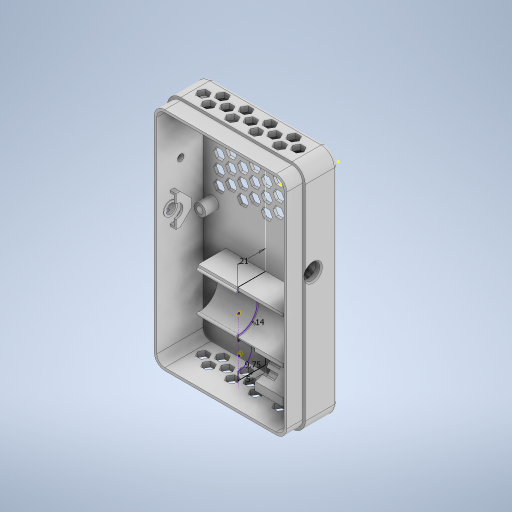
# Autodesk Inventor part: Bottom Housing
Saved by Autodesk Inventor 2023 (Build 270158000, 158)
## iProperties
Created: 2024-03-20
Part Number: Bottom Housing
Material: Generic
Document SubType Name: Modeling
Designer: Pobe Tran
Density: 1 g/cm^3
Appearance: Default
Author: Pobe Tran
Autodesk Inventor part; units mm, degrees
(part 1 of 2)
sketch "Sketch2" plane through (0, 0, 0) normal (0, 0, 1) x (1, 0, 0)
  line L0 (0, 0) -> (-90.043, 0)
  line L1 (-90.043, 0) -> (-90.043, -76.2)
  line L2 (-90.043, -76.2) -> (0, -76.2)
  line L3 (0, -76.2) -> (0, 0)
  circle A0 centre (-6.858, -17.272) radius 0.45
  circle A1 centre (-11.938, -17.272) radius 0.45
  circle A2 centre (-9.398, -17.272) radius 0.45
  circle A3 centre (-9.398, -35.052) radius 0.45
  circle A4 centre (-6.858, -35.052) radius 0.45
  circle A5 centre (-14.478, -17.272) radius 0.45
  circle A6 centre (-14.478, -35.052) radius 0.45
  circle A7 centre (-17.018, -17.272) radius 0.45
  circle A8 centre (-22.098, -17.272) radius 0.45
  circle A9 centre (-19.558, -17.272) radius 0.45
  circle A10 centre (-27.178, -17.272) radius 0.45
  circle A11 centre (-24.638, -17.272) radius 0.45
  circle A12 centre (-29.718, -17.272) radius 0.45
  circle A13 centre (-29.718, -35.052) radius 0.45
  circle A14 centre (-4.445, -46.736) radius 0.55
  circle A15 centre (-11.938, -35.052) radius 0.45
  circle A16 centre (-4.445, -44.196) radius 0.55
  circle A17 centre (-4.445, -49.276) radius 0.55
  line L4 (-11.023, -61.594) -> (-11.023, -64.644)
  line L5 (-10.263, -61.594) -> (-11.023, -61.594)
  line L6 (-10.263, -64.644) -> (-10.263, -61.594)
  line L7 (-11.023, -64.644) -> (-10.263, -64.644)
  line L8 (-14.498, -58.009) -> (-14.498, -58.769)
  line L9 (-11.448, -58.009) -> (-14.498, -58.009)
  line L10 (-11.448, -58.769) -> (-11.448, -58.009)
  line L11 (-14.498, -58.769) -> (-11.448, -58.769)
  line L12 (-16.953, -61.594) -> (-16.953, -64.644)
  line L13 (-16.193, -61.594) -> (-16.953, -61.594)
  line L14 (-16.193, -64.644) -> (-16.193, -61.594)
  line L15 (-16.953, -64.644) -> (-16.193, -64.644)
  circle A18 centre (-17.018, -35.052) radius 0.45
  circle A19 centre (-22.098, -35.052) radius 0.45
  circle A20 centre (-19.558, -35.052) radius 0.45
  circle A21 centre (-27.178, -35.052) radius 0.45
  circle A22 centre (-24.638, -35.052) radius 0.45
  circle A23 centre (-28.067, -58.036) radius 0.35
  circle A24 centre (-28.067, -65.662) radius 0.35
  circle A25 centre (-32.258, -17.272) radius 0.45
  circle A26 centre (-37.338, -17.272) radius 0.45
  circle A27 centre (-34.798, -17.272) radius 0.45
  circle A28 centre (-37.338, -35.052) radius 0.45
  circle A29 centre (-32.258, -35.052) radius 0.45
  circle A30 centre (-39.878, -17.272) radius 0.45
  circle A31 centre (-39.878, -35.052) radius 0.45
  circle A32 centre (-42.418, -17.272) radius 0.45
  circle A33 centre (-47.498, -17.272) radius 0.45
  circle A34 centre (-44.958, -17.272) radius 0.45
  circle A35 centre (-52.578, -17.272) radius 0.45
  circle A36 centre (-50.038, -17.272) radius 0.45
  circle A37 centre (-55.118, -17.272) radius 0.45
  circle A38 centre (-52.578, -35.052) radius 0.45
  circle A39 centre (-34.798, -35.052) radius 0.45
  circle A40 centre (-44.958, -35.052) radius 0.45
  circle A41 centre (-42.418, -35.052) radius 0.45
  circle A42 centre (-32.893, -61.595) radius 0.55
  circle A43 centre (-32.893, -64.135) radius 0.55
  circle A44 centre (-46.101, -58.036) radius 0.35
  circle A45 centre (-32.893, -59.055) radius 0.55
  circle A46 centre (-47.498, -35.052) radius 0.45
  circle A47 centre (-45.212, -46.355) radius 1.9
  circle A48 centre (-55.118, -35.052) radius 0.45
  circle A49 centre (-50.038, -35.052) radius 0.45
  circle A50 centre (-50.546, -64.135) radius 0.55
  circle A51 centre (-46.101, -65.662) radius 0.35
  circle A52 centre (-50.546, -59.055) radius 0.55
  circle A53 centre (-50.546, -61.595) radius 0.55
  line L16 (-93.5594, -83.82) -> (-93.5594, 3.4535)
  line L17 (-93.5594, 3.4535) -> (2.8371, 3.4535)
  line L18 (2.8371, 3.4535) -> (2.8371, -113.1572)
  line L19 (2.8371, -113.1572) -> (2.8371, -163.9139)
  line L20 (2.8371, -163.9139) -> (-93.5594, -163.9139)
  line L21 (-93.5594, -163.9139) -> (-93.5594, -83.82)
  constraints: 54 centre point, 44 end point, 2 collinear
extrude "Extrusion2" add sketch "Sketch2" along normal blind 2 contours L3 L2 L1 L0 | A0 | A1 | A2 | A3 | A4 | A5 | A6 | A7 | A8 | A9 | A10 | A11 | A12 | A13 | A14 | A15 | A16 | A17 | L5 L6 L7 L4 | L9 L10 L11 L8 | L13 L14 L15 L12 | A18 | A19 | A20 | A21 | A22 | A23 | A24 | A25 | A26 | A27 | A28 | A29 | A30 | A31 | A32 | A33 | A34 | A35 | A36 | A37 | A38 | A39 | A40 | A41 | A42 | A43 | A44 | A45 | A46 | A47 | A48 | A49 | A50 | A51 | A52 | A53 | L16 L17 L18 L19 L20 L21
sketch "Sketch3" plane through (0, 0, 2) normal (0, 0, 1) x (1, 0, 0)
  line L0 (-90.043, 0) -> (-90.043, -76.2) projected
  line L1 (-90.043, -76.2) -> (0, -76.2) projected
  line L2 (0, -76.2) -> (0, 0) projected
  line L3 (0, 0) -> (-90.043, 0) projected
  circle A0 centre (-4, -72.2) radius 2.45
  circle A1 centre (-4, -4) radius 2.45
  circle A2 centre (-86.043, -72.2) radius 2.45
  circle A3 centre (-86.043, -4) radius 2.45
  circle A4 centre (-4, -72.2) radius 4.45
  circle A5 centre (-86.043, -72.2) radius 4.45
  circle A6 centre (-4, -4) radius 4.45
  circle A7 centre (-86.043, -4) radius 4.45
  dimension "d8" = 4
  dimension "d9" = 4
  dimension "d14" = 4
  dimension "d15" = 4
  dimension "d16" = 4.9
  dimension "d17" = 4.9
  dimension "d18" = 4.9
  dimension "d19" = 4.9
  dimension "d22" = 2
  dimension "d23" = 2
  dimension "d24" = 2
  dimension "d25" = 2
  constraints: 8 centre point, 4 coincident, 2 horizontal alignment, 2 vertical alignment
  measures "d8" distance from line of point (-4, -4) L2
  measures "d9" distance from line of point (-4, -4) L3
  measures "d14" distance from line of point (-4, -72.2) L1
  measures "d15" distance from line of L0 point (-86.043, -72.2)
  measures "d16" diameter of A0
  measures "d17" diameter of A1
  measures "d18" diameter of A2
  measures "d19" diameter of A3
  measures "d22" radial gap between concentric circles of A0 A4
  measures "d23" radial gap between concentric circles of A2 A5
  measures "d24" radial gap between concentric circles of A1 A6
  measures "d25" radial gap between concentric circles of A3 A7
extrude "Extrusion4" add sketch "Sketch3" along normal blind 10 contours A7 L3 L0 | L0 A7 | A7 L3 | A5 L1 L0 | L0 A5 | A6 L3 | L3 A6 L2 | L2 A6 | L1 A5 | A4 L2 | L2 A4 L1 | L1 A4 picked at (-86.1414, -0.5226) picked at (-85.9446, -75.6774) picked at (-3.9016, -0.5226) picked at (-3.9016, -75.6774)
sketch "Sketch4" plane through (0, 0, 2) normal (0, 0, 1) x (1, 0, 0)
  point P0 (0, 0)
sketch "Sketch5" plane through (0, 0, 2) normal (0, 0, 1) x (1, 0, 0)
  line L0 (-20.397, -28.9385) -> (-16.0669, -28.9385)
  line L1 (-16.0669, -28.9385) -> (-13.9018, -32.6885)
  line L2 (-13.9018, -32.6885) -> (-16.0669, -36.4385)
  line L3 (-16.0669, -36.4385) -> (-20.397, -36.4385)
  line L4 (-20.397, -36.4385) -> (-22.5621, -32.6885)
  line L5 (-22.5621, -32.6885) -> (-20.397, -28.9385)
  line L6 (-11.397, -34.35) -> (-7.0669, -34.35)
  line L7 (-7.0669, -34.35) -> (-4.9018, -38.1)
  line L8 (-4.9018, -38.1) -> (-7.0669, -41.85)
  line L9 (-7.0669, -41.85) -> (-11.397, -41.85)
  line L10 (-11.397, -41.85) -> (-13.5621, -38.1)
  line L11 (-13.5621, -38.1) -> (-11.397, -34.35)
  line L12 (-20.397, -18.1154) -> (-16.0669, -18.1154)
  line L13 (-16.0669, -18.1154) -> (-13.9018, -21.8654)
  line L14 (-13.9018, -21.8654) -> (-16.0669, -25.6154)
  line L15 (-16.0669, -25.6154) -> (-20.397, -25.6154)
  line L16 (-20.397, -25.6154) -> (-22.5621, -21.8654)
  line L17 (-22.5621, -21.8654) -> (-20.397, -18.1154)
  line L18 (-11.397, -23.5269) -> (-7.0669, -23.5269)
  line L19 (-7.0669, -23.5269) -> (-4.9018, -27.2769)
  line L20 (-4.9018, -27.2769) -> (-7.0669, -31.0269)
  line L21 (-7.0669, -31.0269) -> (-11.397, -31.0269)
  line L22 (-11.397, -31.0269) -> (-13.5621, -27.2769)
  line L23 (-13.5621, -27.2769) -> (-11.397, -23.5269)
  line L24 (-31.5621, -27.2769) -> (-29.397, -23.5269)
  line L25 (-29.397, -23.5269) -> (-25.0669, -23.5269)
  line L26 (-25.0669, -23.5269) -> (-22.9018, -27.2769)
  line L27 (-29.397, -31.0269) -> (-31.5621, -27.2769)
  line L28 (-22.9018, -27.2769) -> (-25.0669, -31.0269)
  line L29 (-25.0669, -31.0269) -> (-29.397, -31.0269)
  line L30 (-29.397, -34.35) -> (-25.0669, -34.35)
  line L31 (-31.5621, -38.1) -> (-29.397, -34.35)
  line L32 (-29.397, -41.85) -> (-31.5621, -38.1)
  line L33 (-25.0669, -34.35) -> (-22.9018, -38.1)
  line L34 (-25.0669, -41.85) -> (-29.397, -41.85)
  line L35 (-22.9018, -38.1) -> (-25.0669, -41.85)
  line L36 (-38.397, -28.9385) -> (-34.0669, -28.9385)
  line L37 (-34.0669, -28.9385) -> (-31.9018, -32.6885)
  line L38 (-31.9018, -32.6885) -> (-34.0669, -36.4385)
  line L39 (-34.0669, -36.4385) -> (-38.397, -36.4385)
  line L40 (-38.397, -36.4385) -> (-40.5621, -32.6885)
  line L41 (-40.5621, -32.6885) -> (-38.397, -28.9385)
  line L42 (-34.0669, -25.6154) -> (-38.397, -25.6154)
  line L43 (-31.9018, -21.8654) -> (-34.0669, -25.6154)
  line L44 (-34.0669, -18.1154) -> (-31.9018, -21.8654)
  line L45 (-38.397, -25.6154) -> (-40.5621, -21.8654)
  line L46 (-38.397, -18.1154) -> (-34.0669, -18.1154)
  line L47 (-40.5621, -21.8654) -> (-38.397, -18.1154)
  line L48 (-20.397, -50.2615) -> (-16.0669, -50.2615)
  line L49 (-16.0669, -50.2615) -> (-13.9018, -54.0115)
  line L50 (-13.9018, -54.0115) -> (-16.0669, -57.7615)
  line L51 (-16.0669, -57.7615) -> (-20.397, -57.7615)
  line L52 (-20.397, -57.7615) -> (-22.5621, -54.0115)
  line L53 (-22.5621, -54.0115) -> (-20.397, -50.2615)
  line L54 (-11.397, -55.6731) -> (-7.0669, -55.6731)
  line L55 (-7.0669, -55.6731) -> (-4.9018, -59.4231)
  line L56 (-4.9018, -59.4231) -> (-7.0669, -63.1731)
  line L57 (-7.0669, -63.1731) -> (-11.397, -63.1731)
  line L58 (-11.397, -63.1731) -> (-13.5621, -59.4231)
  line L59 (-13.5621, -59.4231) -> (-11.397, -55.6731)
  line L60 (-20.397, -39.4385) -> (-16.0669, -39.4385)
  line L61 (-16.0669, -39.4385) -> (-13.9018, -43.1885)
  line L62 (-13.9018, -43.1885) -> (-16.0669, -46.9385)
  line L63 (-16.0669, -46.9385) -> (-20.397, -46.9385)
  line L64 (-20.397, -46.9385) -> (-22.5621, -43.1885)
  line L65 (-22.5621, -43.1885) -> (-20.397, -39.4385)
  line L66 (-11.397, -44.85) -> (-7.0669, -44.85)
  line L67 (-7.0669, -44.85) -> (-4.9018, -48.6)
  line L68 (-4.9018, -48.6) -> (-7.0669, -52.35)
  line L69 (-7.0669, -52.35) -> (-11.397, -52.35)
  line L70 (-11.397, -52.35) -> (-13.5621, -48.6)
  line L71 (-13.5621, -48.6) -> (-11.397, -44.85)
  line L72 (-31.5621, -48.6) -> (-29.397, -44.85)
  line L73 (-29.397, -44.85) -> (-25.0669, -44.85)
  line L74 (-25.0669, -44.85) -> (-22.9018, -48.6)
  line L75 (-29.397, -52.35) -> (-31.5621, -48.6)
  line L76 (-22.9018, -48.6) -> (-25.0669, -52.35)
  line L77 (-25.0669, -52.35) -> (-29.397, -52.35)
  line L78 (-29.397, -55.6731) -> (-25.0669, -55.6731)
  line L79 (-31.5621, -59.4231) -> (-29.397, -55.6731)
  line L80 (-29.397, -63.1731) -> (-31.5621, -59.4231)
  line L81 (-25.0669, -55.6731) -> (-22.9018, -59.4231)
  line L82 (-25.0669, -63.1731) -> (-29.397, -63.1731)
  line L83 (-22.9018, -59.4231) -> (-25.0669, -63.1731)
  line L84 (-38.397, -50.2615) -> (-34.0669, -50.2615)
  line L85 (-34.0669, -50.2615) -> (-31.9018, -54.0115)
  line L86 (-31.9018, -54.0115) -> (-34.0669, -57.7615)
  line L87 (-34.0669, -57.7615) -> (-38.397, -57.7615)
  line L88 (-38.397, -57.7615) -> (-40.5621, -54.0115)
  line L89 (-40.5621, -54.0115) -> (-38.397, -50.2615)
  line L90 (-34.0669, -46.9385) -> (-38.397, -46.9385)
  line L91 (-31.9018, -43.1885) -> (-34.0669, -46.9385)
  line L92 (-34.0669, -39.4385) -> (-31.9018, -43.1885)
  line L93 (-38.397, -46.9385) -> (-40.5621, -43.1885)
  line L94 (-38.397, -39.4385) -> (-34.0669, -39.4385)
  line L95 (-40.5621, -43.1885) -> (-38.397, -39.4385)
  line L96 (-36.232, -21.8654) -> (-36.232, -54.0115) construction
  line L97 (-52.0669, -28.9385) -> (-56.397, -28.9385)
  line L98 (-56.397, -28.9385) -> (-58.5621, -32.6885)
  line L99 (-58.5621, -32.6885) -> (-56.397, -36.4385)
  line L100 (-56.397, -36.4385) -> (-52.0669, -36.4385)
  line L101 (-52.0669, -36.4385) -> (-49.9018, -32.6885)
  line L102 (-49.9018, -32.6885) -> (-52.0669, -28.9385)
  line L103 (-61.0669, -34.35) -> (-65.397, -34.35)
  line L104 (-65.397, -34.35) -> (-67.5621, -38.1)
  line L105 (-67.5621, -38.1) -> (-65.397, -41.85)
  line L106 (-65.397, -41.85) -> (-61.0669, -41.85)
  line L107 (-61.0669, -41.85) -> (-58.9018, -38.1)
  line L108 (-58.9018, -38.1) -> (-61.0669, -34.35)
  line L109 (-52.0669, -18.1154) -> (-56.397, -18.1154)
  line L110 (-56.397, -18.1154) -> (-58.5621, -21.8654)
  line L111 (-58.5621, -21.8654) -> (-56.397, -25.6154)
  line L112 (-56.397, -25.6154) -> (-52.0669, -25.6154)
  line L113 (-52.0669, -25.6154) -> (-49.9018, -21.8654)
  line L114 (-49.9018, -21.8654) -> (-52.0669, -18.1154)
  line L115 (-61.0669, -23.5269) -> (-65.397, -23.5269)
  line L116 (-65.397, -23.5269) -> (-67.5621, -27.2769)
  line L117 (-67.5621, -27.2769) -> (-65.397, -31.0269)
  line L118 (-65.397, -31.0269) -> (-61.0669, -31.0269)
  line L119 (-61.0669, -31.0269) -> (-58.9018, -27.2769)
  line L120 (-58.9018, -27.2769) -> (-61.0669, -23.5269)
  line L121 (-40.9018, -27.2769) -> (-43.0669, -23.5269)
  line L122 (-43.0669, -23.5269) -> (-47.397, -23.5269)
  line L123 (-47.397, -23.5269) -> (-49.5621, -27.2769)
  line L124 (-43.0669, -31.0269) -> (-40.9018, -27.2769)
  line L125 (-49.5621, -27.2769) -> (-47.397, -31.0269)
  line L126 (-47.397, -31.0269) -> (-43.0669, -31.0269)
  line L127 (-43.0669, -34.35) -> (-47.397, -34.35)
  line L128 (-40.9018, -38.1) -> (-43.0669, -34.35)
  line L129 (-43.0669, -41.85) -> (-40.9018, -38.1)
  line L130 (-47.397, -34.35) -> (-49.5621, -38.1)
  line L131 (-47.397, -41.85) -> (-43.0669, -41.85)
  line L132 (-49.5621, -38.1) -> (-47.397, -41.85)
  line L133 (-52.0669, -50.2615) -> (-56.397, -50.2615)
  line L134 (-56.397, -50.2615) -> (-58.5621, -54.0115)
  line L135 (-65.397, -52.35) -> (-61.0669, -52.35)
  line L136 (-61.0669, -52.35) -> (-58.9018, -48.6)
  line L137 (-67.5621, -48.6) -> (-65.397, -52.35)
  line L138 (-65.397, -44.85) -> (-67.5621, -48.6)
  line L139 (-61.0669, -44.85) -> (-65.397, -44.85)
  line L140 (-58.9018, -48.6) -> (-61.0669, -44.85)
  line L141 (-56.397, -46.9385) -> (-52.0669, -46.9385)
  line L142 (-58.5621, -43.1885) -> (-56.397, -46.9385)
  line L143 (-52.0669, -39.4385) -> (-56.397, -39.4385)
  line L144 (-56.397, -39.4385) -> (-58.5621, -43.1885)
  line L145 (-43.0669, -52.35) -> (-40.9018, -48.6)
  line L146 (-40.9018, -48.6) -> (-43.0669, -44.85)
  line L147 (-43.0669, -55.6731) -> (-47.397, -55.6731)
  line L148 (-47.397, -52.35) -> (-43.0669, -52.35)
  line L149 (-43.0669, -44.85) -> (-47.397, -44.85)
  line L150 (-47.397, -44.85) -> (-49.5621, -48.6)
  line L151 (-49.5621, -48.6) -> (-47.397, -52.35)
  line L152 (-49.9018, -54.0115) -> (-52.0669, -50.2615)
  line L153 (-52.0669, -57.7615) -> (-49.9018, -54.0115)
  line L154 (-52.0669, -46.9385) -> (-49.9018, -43.1885)
  line L155 (-49.9018, -43.1885) -> (-52.0669, -39.4385)
  line L156 (-58.5621, -54.0115) -> (-56.397, -57.7615)
  line L157 (-56.397, -57.7615) -> (-52.0669, -57.7615)
  line L158 (-61.0669, -55.6731) -> (-65.397, -55.6731)
  line L159 (-58.9018, -59.4231) -> (-61.0669, -55.6731)
  line L160 (-61.0669, -63.1731) -> (-58.9018, -59.4231)
  line L161 (-65.397, -55.6731) -> (-67.5621, -59.4231)
  line L162 (-65.397, -63.1731) -> (-61.0669, -63.1731)
  line L163 (-67.5621, -59.4231) -> (-65.397, -63.1731)
  line L164 (-40.9018, -59.4231) -> (-43.0669, -55.6731)
  line L165 (-47.397, -55.6731) -> (-49.5621, -59.4231)
  line L166 (-47.397, -63.1731) -> (-43.0669, -63.1731)
  line L167 (-49.5621, -59.4231) -> (-47.397, -63.1731)
  line L168 (-43.0669, -63.1731) -> (-40.9018, -59.4231)
  line L169 (-63.232, -27.2769) -> (-63.232, -59.4231) construction
  line L170 (-70.0669, -39.4385) -> (-67.9018, -43.1885)
  line L171 (-67.9018, -32.6885) -> (-70.0669, -36.4385)
  line L172 (-74.397, -39.4385) -> (-70.0669, -39.4385)
  line L173 (-70.0669, -36.4385) -> (-74.397, -36.4385)
  line L174 (-74.397, -36.4385) -> (-76.5621, -32.6885)
  line L175 (-76.5621, -43.1885) -> (-74.397, -39.4385)
  line L176 (-67.9018, -43.1885) -> (-70.0669, -46.9385)
  line L177 (-70.0669, -46.9385) -> (-74.397, -46.9385)
  line L178 (-74.397, -50.2615) -> (-70.0669, -50.2615)
  line L179 (-70.0669, -50.2615) -> (-67.9018, -54.0115)
  line L180 (-74.397, -28.9385) -> (-70.0669, -28.9385)
  line L181 (-70.0669, -28.9385) -> (-67.9018, -32.6885)
  line L182 (-76.5621, -32.6885) -> (-74.397, -28.9385)
  line L183 (-74.397, -18.1154) -> (-70.0669, -18.1154)
  line L184 (-70.0669, -18.1154) -> (-67.9018, -21.8654)
  line L185 (-67.9018, -21.8654) -> (-70.0669, -25.6154)
  line L186 (-70.0669, -25.6154) -> (-74.397, -25.6154)
  line L187 (-74.397, -25.6154) -> (-76.5621, -21.8654)
  line L188 (-76.5621, -21.8654) -> (-74.397, -18.1154)
  line L189 (-74.397, -46.9385) -> (-76.5621, -43.1885)
  line L190 (-76.5621, -54.0115) -> (-74.397, -50.2615)
  line L191 (-70.0669, -57.7615) -> (-74.397, -57.7615)
  line L192 (-67.9018, -54.0115) -> (-70.0669, -57.7615)
  line L193 (-74.397, -57.7615) -> (-76.5621, -54.0115)
  line L194 (-76.9018, -38.1) -> (-79.0669, -41.85)
  line L195 (-79.0669, -34.35) -> (-76.9018, -38.1)
  line L196 (-76.9018, -27.2769) -> (-79.0669, -31.0269)
  line L197 (-83.397, -23.5269) -> (-79.0669, -23.5269)
  line L198 (-79.0669, -31.0269) -> (-83.397, -31.0269)
  line L199 (-85.5621, -27.2769) -> (-83.397, -23.5269)
  line L200 (-83.397, -31.0269) -> (-85.5621, -27.2769)
  line L201 (-83.397, -34.35) -> (-79.0669, -34.35)
  line L202 (-85.5621, -38.1) -> (-83.397, -34.35)
  line L203 (-83.397, -41.85) -> (-85.5621, -38.1)
  line L204 (-79.0669, -23.5269) -> (-76.9018, -27.2769)
  line L205 (-79.0669, -41.85) -> (-83.397, -41.85)
  line L206 (-79.0669, -44.85) -> (-76.9018, -48.6)
  line L207 (-76.9018, -48.6) -> (-79.0669, -52.35)
  line L208 (-83.397, -44.85) -> (-79.0669, -44.85)
  line L209 (-79.0669, -52.35) -> (-83.397, -52.35)
  line L210 (-85.5621, -48.6) -> (-83.397, -44.85)
  line L211 (-83.397, -52.35) -> (-85.5621, -48.6)
  line L212 (-76.9018, -59.4231) -> (-79.0669, -63.1731)
  line L213 (-79.0669, -55.6731) -> (-76.9018, -59.4231)
  line L214 (-83.397, -55.6731) -> (-79.0669, -55.6731)
  line L215 (-85.5621, -59.4231) -> (-83.397, -55.6731)
  line L216 (-83.397, -63.1731) -> (-85.5621, -59.4231)
  line L217 (-79.0669, -63.1731) -> (-83.397, -63.1731)
  line L218 (-72.232, -21.8654) -> (-18.232, -21.8654) construction
  line L219 (-11.397, -20.2038) -> (-7.0669, -20.2038)
  line L220 (-7.0669, -20.2038) -> (-4.9018, -16.4538)
  line L221 (-4.9018, -16.4538) -> (-7.0669, -12.7038)
  line L222 (-7.0669, -12.7038) -> (-11.397, -12.7038)
  line L223 (-11.397, -12.7038) -> (-13.5621, -16.4538)
  line L224 (-13.5621, -16.4538) -> (-11.397, -20.2038)
  line L225 (-31.5621, -16.4538) -> (-29.397, -20.2038)
  line L226 (-29.397, -20.2038) -> (-25.0669, -20.2038)
  line L227 (-25.0669, -20.2038) -> (-22.9018, -16.4538)
  line L228 (-29.397, -12.7038) -> (-31.5621, -16.4538)
  line L229 (-22.9018, -16.4538) -> (-25.0669, -12.7038)
  line L230 (-25.0669, -12.7038) -> (-29.397, -12.7038)
  line L231 (-49.5621, -16.4538) -> (-47.397, -12.7038)
  line L232 (-43.0669, -20.2038) -> (-47.397, -20.2038)
  line L233 (-47.397, -12.7038) -> (-43.0669, -12.7038)
  line L234 (-40.9018, -16.4538) -> (-43.0669, -20.2038)
  line L235 (-43.0669, -12.7038) -> (-40.9018, -16.4538)
  line L236 (-47.397, -20.2038) -> (-49.5621, -16.4538)
  line L237 (-61.0669, -12.7038) -> (-58.9018, -16.4538)
  line L238 (-58.9018, -16.4538) -> (-61.0669, -20.2038)
  line L239 (-65.397, -12.7038) -> (-61.0669, -12.7038)
  line L240 (-61.0669, -20.2038) -> (-65.397, -20.2038)
  line L241 (-65.397, -20.2038) -> (-67.5621, -16.4538)
  line L242 (-67.5621, -16.4538) -> (-65.397, -12.7038)
  line L243 (-63.232, -16.4538) -> (-63.232, 15.6923) construction
  line L244 (-79.0669, -20.2038) -> (-76.9018, -16.4538)
  line L245 (-76.9018, -16.4538) -> (-79.0669, -12.7038)
  line L246 (-83.397, -20.2038) -> (-79.0669, -20.2038)
  line L247 (-85.5621, -16.4538) -> (-83.397, -20.2038)
  line L248 (-83.397, -12.7038) -> (-85.5621, -16.4538)
  line L249 (-79.0669, -12.7038) -> (-83.397, -12.7038)
  line L250 (-81.232, -38.1) -> (-9.232, -38.1) construction
  circle A0 centre (-86.043, -4) radius 2.45 construction
  circle A1 centre (-86.043, -72.2) radius 2.45 construction
  line L251 (-86.043, -4) -> (-86.043, -72.2) construction
  line L252 (-86.043, -4) -> (-4.4209, -4) construction
  line L253 (-45.232, -16.4538) -> (-45.232, -59.4231) construction
  point P0 (0, 0)
  point P1 (-18.232, -32.6885)
  point P2 (-9.232, -27.2769)
  point P3 (-27.232, -38.1)
  point P4 (-27.232, -27.2769)
  point P5 (-36.232, -32.6885)
  point P6 (-18.232, -54.0115)
  point P7 (-9.232, -59.4231)
  point P8 (-18.232, -43.1885)
  point P9 (-9.232, -48.6)
  point P10 (-27.232, -59.4231)
  point P11 (-27.232, -48.6)
  point P12 (-36.232, -43.1885)
  point P13 (-54.232, -32.6885)
  point P14 (-63.232, -38.1)
  point P15 (-54.232, -21.8654)
  point P16 (-45.232, -38.1)
  point P17 (-45.232, -27.2769)
  point P18 (-63.232, -48.6)
  point P19 (-54.232, -43.1885)
  point P20 (-45.232, -48.6)
  point P21 (-54.232, -54.0115)
  point P22 (-72.232, -43.1885)
  point P23 (-72.232, -32.6885)
  point P24 (-72.232, -54.0115)
  point P25 (-81.232, -27.2769)
  point P26 (-81.232, -48.6)
  point P27 (-81.232, -59.4231)
  point P28 (-9.232, -16.4538)
  point P29 (-27.232, -16.4538)
  point P30 (-81.232, -16.4538)
  point P31 (-86.043, -38.1)
  point P32 (-45.232, -4)
  dimension "d28" = 7.5
  dimension "d29" = 7.5
  dimension "d30" = 3
  dimension "d31" = 7.5
  dimension "d32" = 7.5
  dimension "d33" = 3
  dimension "d34" = 3
  dimension "d37" = 18
  dimension "d42" = 3
  dimension "d43" = 3
  dimension "d48" = 7.5
  dimension "d49" = 7.5
  dimension "d50" = 3
  dimension "d51" = 7.5
  dimension "d52" = 7.5
  dimension "d53" = 3
  dimension "d54" = 3
  dimension "d55" = 18
  dimension "d56" = 3
  dimension "d57" = 3
  dimension "d59" = 3
  constraints: 508 end point, 176 symmetric about line, 4 vertical alignment, 3 horizontal, 2 collinear, 2 midpoint, 2 vertical, 206 other
  measures "d28" distance between parallel lines of L0 L3
  measures "d29" distance between parallel lines of L6 L9
  measures "d30" distance between parallel lines of L2 L11
  measures "d31" distance between parallel lines of L12 L15
  measures "d32" distance between parallel lines of L18 L21
  measures "d33" distance between parallel lines of L14 L23
  measures "d34" distance between parallel lines of L22 L1
  measures "d37" distance of L250.end point (-27.232, -38.1)
  measures "d42" distance between parallel lines of L5 L28
  measures "d43" distance between parallel lines of L4 L33
  measures "d48" distance between parallel lines of L48 L51
  measures "d49" distance between parallel lines of L54 L57
  measures "d50" distance between parallel lines of L50 L59
  measures "d51" distance between parallel lines of L60 L63
  measures "d52" distance between parallel lines of L66 L69
  measures "d53" distance between parallel lines of L62 L71
  measures "d54" distance between parallel lines of L70 L49
  measures "d55" distance of point (-9.232, -59.423) point (-27.232, -59.423)
  measures "d56" distance between parallel lines of L53 L76
  measures "d57" distance between parallel lines of L52 L81
  measures "d59" distance of L67.start L8.end
extrude "Extrusion5" cut sketch "Sketch5" against normal through all
ref_plane "Work Plane5" through (-18.3368, -95.497, 22.3224) normal (1, 0, 0) x (0, -0.4604848, 0.8876676)
sketch "Sketch7" plane through (-18.3368, -95.497, 22.3224) normal (1, 0, 0) x (0, -0.4604848, 0.8876676)
  line L0 (-63.6047, -78.477) -> (13.4654, 70.0896) projected
  line L1 (-11.115, 22.7064) -> (-25.6416, -5.2963)
  line L2 (-11.115, 22.7064) -> (-25.3738, -4.78)
  line L3 (13.4654, 70.0896) -> (-63.6047, -78.477) projected
  line L4 (17.6699, 32.5904) -> (-0.9711, 42.2606)
  line L5 (-11.115, 22.7064) -> (-9.776, 25.2876)
  line L6 (1.5185, 1.4556) -> (-17.1225, 11.1258)
  line L7 (-25.3738, -4.78) -> (-17.1225, 11.1258)
  arc A0 (16.6327, 30.591) -> (2.5557, 3.455) centre (8.9927, 17.335) ccw
  line L8 (1.5185, 1.4556) -> (2.5557, 3.455)
  line L9 (11.6901, 71.0106) -> (13.4654, 70.0896) projected
  line L10 (17.6699, 32.5904) -> (16.6327, 30.591)
  line L11 (8.9927, 17.335) -> (14.927, 28.7745) construction
  circle A1 centre (8.9927, 17.335) radius 1.5875 projected
  circle A2 centre (8.9927, 17.335) radius 15.3 projected
  circle A3 centre (8.9927, 17.335) radius 14 projected
  point P0 (-63.7898, -74.4905)
  point P1 (22.9456, 11.0577)
  point P2 (22.1601, 9.5434)
  point P3 (-21.2482, 3.1729)
  point P4 (-17.1225, 11.1258)
  point P5 (-0.9711, 42.2606)
  point P6 (12.5777, 70.5501)
  dimension "d71" = 35.0748
  dimension "d159" = 15.3
  dimension "d160" = 21
  constraints: 18 end point, 7 point on line, 4 point on circle, 3 parallel, 2 equal length, 2 midpoint, 2 perpendicular, 1 centre point, 1 collinear
  measures "d71" distance between parallel lines of L6 L4
  measures "d159" radius of A0
  measures "d160" distance between parallel lines of L2 L8
extrude "Extrusion6" add sketch "Sketch7" along normal blind 5 and the other way blind 28 contours L0 L4 L10 A0 L8 L6
sketch "Sketch8" plane through (-46.3368, -95.497, 22.3224) normal (-1, 0, 0) x (0, -0.4604848, 0.8876676)
  line L0 (-63.6047, 78.477) -> (13.4654, -70.0896) projected
  line L1 (3.1465, -4.5939) -> (1.5185, -1.4556)
  line L2 (-17.1225, -11.1258) -> (1.5185, -1.4556) projected
  line L3 (1.5185, -1.4556) -> (-17.1225, -11.1258)
  line L4 (-17.1225, -11.1258) -> (11.163, -65.6513)
  arc A0 (3.1465, -4.5939) -> (16.0254, -29.4204) centre (8.9946, -17.3139) ccw
  line L5 (29.804, -55.9811) -> (11.163, -65.6513)
  line L6 (16.0254, -29.4204) -> (18.0003, -33.2273)
  line L7 (26.9588, -50.4963) -> (29.804, -55.9811)
  arc A1 (18.0003, -33.2273) -> (26.9588, -50.4963) centre (21.8882, -42.1686) ccw
  line L8 (11.6901, -71.0106) -> (13.4654, -70.0896) projected
  line L9 (8.9946, -17.3139) -> (32.3631, -62.3609) construction
  line L10 (16.6327, -30.591) -> (17.6699, -32.5904) projected
  line L11 (17.6699, -32.5904) -> (-0.9711, -42.2606)
  line L12 (17.0129, -31.3238) -> (-1.6282, -40.994)
  circle A2 centre (8.9927, -17.335) radius 1.5875 projected
  ellipse E0 centre (20.7156, -41.9283) end of major axis (20.2797, -43.8802) minor radius 1.9704 projected
  point P0 (-63.7898, 74.4905)
  point P1 (2.8668, -43.144)
  point P2 (-1.6282, -40.994)
  dimension "d79" = 21
  dimension "d161" = 5
  dimension "d162" = 9.75
  dimension "d163" = 14
  constraints: 19 end point, 6 point on line, 4 parallel, 4 point on circle, 3 perpendicular, 2 centre point, 1 coincident, 1 collinear, 1 midpoint, 1 other
  measures "d79" distance between parallel lines of L0 L1
  measures "d161" distance between parallel lines of L5 L8
  measures "d162" radius of A1
  measures "d163" radius of A0
extrude "Extrusion7" add sketch "Sketch8" along normal blind 30 contours L2 L1 A0 L6 L12 L0
sketch "Sketch11" plane through (0, 0, 2) normal (0, 0, 1) x (1, 0, 0)
  line L0 (-93.5594, 3.4535) -> (-93.5594, -163.9139) projected
  line L1 (-87.5594, -167.9139) -> (-3.1629, -167.9139)
  line L2 (6.8371, -157.9139) -> (6.8371, -2.5465)
  line L3 (-3.1629, 7.4535) -> (-87.5594, 7.4535)
  line L4 (-97.5594, -2.5465) -> (-97.5594, -157.9139)
  arc A0 (-97.5594, -157.9139) -> (-87.5594, -167.9139) centre (-87.5594, -157.9139) ccw
  arc A1 (-87.5594, 7.4535) -> (-97.5594, -2.5465) centre (-87.5594, -2.5465) ccw
  arc A2 (-3.1629, -167.9139) -> (6.8371, -157.9139) centre (-3.1629, -157.9139) ccw
  arc A3 (6.8371, -2.5465) -> (-3.1629, 7.4535) centre (-3.1629, -2.5465) ccw
  line L5 (-93.5594, -19.0465) -> (-93.5594, -141.4139)
  line L6 (2.8371, 3.4535) -> (-93.5594, 3.4535) projected
  line L7 (-93.5594, -163.9139) -> (2.8371, -163.9139) projected
  line L8 (2.8371, -163.9139) -> (2.8371, 3.4535) projected
  line L9 (-93.5594, -157.9139) -> (-93.5594, -2.5465)
  arc A4 (-87.5594, 3.4535) -> (-93.5594, -2.5465) centre (-87.5594, -2.5465) ccw
  line L10 (-87.5594, 3.4535) -> (-3.1629, 3.4535)
  arc A5 (2.8371, -2.5465) -> (-3.1629, 3.4535) centre (-3.1629, -2.5465) ccw
  line L11 (2.8371, -2.5465) -> (2.8371, -157.9139)
  arc A6 (-3.1629, -163.9139) -> (2.8371, -157.9139) centre (-3.1629, -157.9139) ccw
  line L12 (-3.1629, -163.9139) -> (-87.5594, -163.9139)
  arc A7 (-93.5594, -157.9139) -> (-87.5594, -163.9139) centre (-87.5594, -157.9139) ccw
  line L13 (-87.5594, -165.9139) -> (-3.1629, -165.9139)
  arc A8 (-3.1629, -165.9139) -> (4.8371, -157.9139) centre (-3.1629, -157.9139) ccw
  line L14 (4.8371, -157.9139) -> (4.8371, -2.5465)
  arc A9 (4.8371, -2.5465) -> (-3.1629, 5.4535) centre (-3.1629, -2.5465) ccw
  line L15 (-3.1629, 5.4535) -> (-87.5594, 5.4535)
  arc A10 (-87.5594, 5.4535) -> (-95.5594, -2.5465) centre (-87.5594, -2.5465) ccw
  line L16 (-95.5594, -2.5465) -> (-95.5594, -157.9139)
  arc A11 (-95.5594, -157.9139) -> (-87.5594, -165.9139) centre (-87.5594, -157.9139) ccw
  point P0 (-97.5594, -167.9139)
  point P1 (6.8371, -167.9139)
  point P2 (6.8371, 7.4535)
  point P3 (-97.5594, 7.4535)
  point P4 (2.8371, -2.5465)
  point P5 (-3.1629, -163.9139)
  point P6 (-87.5594, 3.4535)
  dimension "d97" = 10
  dimension "d113" = 4
  dimension "d114" = 4
  dimension "d115" = 4
  dimension "d116" = 4
  dimension "d117" = 2
  constraints: 26 end point, 24 point on circle, 12 centre point, 9 point on line, 8 tangent, 6 parallel, 3 equal radius, 3 perpendicular, 14 other
  measures "d97" radius of A0
  measures "d113" distance between parallel lines of L0 L4
  measures "d114" distance between parallel lines of L6 L3
  measures "d115" distance between parallel lines of L1 L7
  measures "d116" distance between parallel lines of L2 L8
  measures "d117" radial gap between concentric circles of A0 A11
extrude "Extrusion10" add sketch "Sketch11" along normal blind 35 and the other way blind 2 contours L0 A11 L16 A10 | L0 A10 L6 A4 | L0 L6 A10 | L6 A10 L15 A9 | L6 A9 L8 A5 | A7 L7 A11 L0 | L6 L8 A9 | L8 A9 L14 A8 | A11 L7 L0 | L7 A8 L13 A11 | L8 A8 L7 A6 | L8 L7 A8 | A0 L4 A1 L3 A3 L2 A2 L1
sketch "Sketch14" plane through (0, 0, 37) normal (0, 0, 1) x (1, 0, 0)
  point P0 (0, 0)
sketch "Sketch15" plane through (0, 0, 37) normal (0, 0, 1) x (1, 0, 0)
  arc A0 (-3.1629, -167.9139) -> (6.8371, -157.9139) centre (-3.1629, -157.9139) ccw projected
  line L0 (6.8371, -157.9139) -> (6.8371, -2.5465) projected
  arc A1 (6.8371, -2.5465) -> (-3.1629, 7.4535) centre (-3.1629, -2.5465) ccw projected
  line L1 (-3.1629, 7.4535) -> (-87.5594, 7.4535) projected
  arc A2 (-87.5594, 7.4535) -> (-97.5594, -2.5465) centre (-87.5594, -2.5465) ccw projected
  line L2 (-97.5594, -2.5465) -> (-97.5594, -157.9139) projected
  arc A3 (-97.5594, -157.9139) -> (-87.5594, -167.9139) centre (-87.5594, -157.9139) ccw projected
  line L3 (-87.5594, -167.9139) -> (-3.1629, -167.9139) projected
  line L4 (2.8371, -2.5465) -> (2.8371, -157.9139) projected
  arc A4 (-3.1629, -163.9139) -> (2.8371, -157.9139) centre (-3.1629, -157.9139) ccw projected
  line L5 (-3.1629, -163.9139) -> (-87.5594, -163.9139) projected
  arc A5 (-93.5594, -157.9139) -> (-87.5594, -163.9139) centre (-87.5594, -157.9139) ccw projected
  line L6 (-93.5594, -157.9139) -> (-93.5594, -2.5465) projected
  arc A6 (-87.5594, 3.4535) -> (-93.5594, -2.5465) centre (-87.5594, -2.5465) ccw projected
  line L7 (-87.5594, 3.4535) -> (-3.1629, 3.4535) projected
  arc A7 (2.8371, -2.5465) -> (-3.1629, 3.4535) centre (-3.1629, -2.5465) ccw projected
  line L8 (4.8371, -2.5465) -> (4.8371, -157.9139)
  arc A8 (-3.1629, -165.9139) -> (4.8371, -157.9139) centre (-3.1629, -157.9139) ccw
  line L9 (-3.1629, -165.9139) -> (-87.5594, -165.9139)
  arc A9 (-95.5594, -157.9139) -> (-87.5594, -165.9139) centre (-87.5594, -157.9139) ccw
  line L10 (-95.5594, -157.9139) -> (-95.5594, -2.5465)
  arc A10 (-87.5594, 5.4535) -> (-95.5594, -2.5465) centre (-87.5594, -2.5465) ccw
  line L11 (-87.5594, 5.4535) -> (-3.1629, 5.4535)
  arc A11 (4.8371, -2.5465) -> (-3.1629, 5.4535) centre (-3.1629, -2.5465) ccw
  point P0 (0, 0)
  dimension "d120" = 2
  constraints: 8 end point, 8 point on circle, 4 centre point, 7 other
  measures "d120" distance between parallel lines of L0 L8
extrude "Extrusion12" cut sketch "Sketch15" against normal blind 12
sketch "Sketch16" plane through (6.8371, -157.9139, 0) normal (1, 0, 0) x (0, 0, -1)
  arc A0 (-19.5791, 99.2547) -> (-18.9791, 90.2949) centre (-18.9791, 94.7949) ccw projected
  arc A1 (-17.7544, 96.0449) -> (-17.7544, 93.5449) centre (-18.9791, 94.7949) ccw projected
  circle A2 centre (-18.9791, 94.7949) radius 6
  point P0 (0, 157.9139)
  dimension "d123" = 12
  constraints: 1 centre point, 1 coincident
  measures "d123" diameter of A2
extrude "Extrusion13" cut sketch "Sketch16" against normal up to next
sketch "Sketch17" plane through (-97.5594, -157.9139, 0) normal (-1, 0, 0) x (0, 0, 1)
  circle A0 centre (18.9791, 119.8139) radius 2.5
  line L0 (12.7191, 157.9139) -> (12.7191, 81.7139) projected
  arc A1 (18.9791, 90.2949) -> (19.5791, 99.2547) centre (18.9791, 94.7949) ccw projected
  point P0 (0, 157.9139)
  point P1 (12.7191, 119.8139)
  dimension "d126" = 5
  constraints: 1 centre point, 1 horizontal alignment, 1 midpoint, 1 vertical alignment
  measures "d126" diameter of A0
extrude "Extrusion14" cut sketch "Sketch17" against normal blind 12
chamfer "Chamfer1" distance 1 angle 45 2 edges at (6.8371, -63.119, 24.9791) (-97.5594, -38.1, 16.4791)
fillet "Fillet2" radius 3 8 edges at (3.9082, -164.985, 0) (-45.3611, -167.9139, 0) (-94.6305, -164.985, 0) (-97.5594, -80.2302, 0) (-94.6305, 4.5245, 0) (-45.3611, 7.4535, 0) (3.9082, 4.5245, 0) (6.8371, -80.2302, 0)
sketch "Sketch18" plane through (6.8371, -157.9139, 25) normal (1, 0, 0) x (0, 0, -1)
  point P0 (25, 157.9139)
ref_plane "Work Plane7" through (-78.0651, -167.9139, 25) normal (1, 0, 0) x (0, 1, 0)
sketch "Sketch24" plane through (-78.0651, -167.9139, 25) normal (1, 0, 0) x (0, 1, 0)
  arc A0 (3.175, 26.5) -> (0, 23.325) centre (3.175, 23.325) ccw projected
  line L0 (36.4678, 24.8) -> (36.4678, 23.5) projected
  line L1 (2, 23.5) -> (36.4678, 23.5) projected
  line L2 (2, 0) -> (2, 23.5) projected
  line L3 (0, 0) -> (2, 0) projected
  line L4 (0, 23.325) -> (0, 0) projected
  line L5 (3.175, 26.5) -> (3.175, 24.8) projected
  line L6 (3.175, 24.8) -> (36.4678, 24.8) projected
  point P0 (167.9139, -25)
ref_plane "Work Plane8" through (-12.439, -167.9139, 25) normal (-1, 0, 0) x (0, 0, 1)
extrude "Extrusion20" [suppressed]
sketch "Sketch25" plane through (-78.0651, -131.4461, 51.5) normal (0, 1, 0) x (1, 0, 0)
  point P0 (78.0651, 51.5)
ref_plane "Work Plane9" through (-69.9262, -125.2739, 49.9384) normal (0, -1, 0) x (1, 0, 0)
sketch "Sketch28" plane through (-46.3368, -95.497, 22.3224) normal (1, 0, 0) x (0, 0.4604848, -0.8876676)
  arc A0 (-26.9588, -50.4963) -> (-18.0003, -33.2273) centre (-21.8882, -42.1686) ccw projected
  line L0 (-17.0129, -31.3238) -> (1.6282, -40.994) projected
  line L1 (-16.0254, -29.4204) -> (-18.0003, -33.2273) projected
  line L2 (63.6047, 78.477) -> (-13.4654, -70.0896) projected
  line L3 (-26.9588, -50.4963) -> (-29.804, -55.9811) projected
  line L4 (-29.804, -55.9811) -> (-11.163, -65.6513) projected
  point P0 (63.7898, 74.4905)
extrude "Extrusion24" add sketch "Sketch28" along normal up to surface (33 mm away)
sketch "Sketch29" plane through (-46.3368, -95.497, 22.3224) normal (-1, 0, 0) x (0, -0.4604848, 0.8876676)
  arc A0 (22.785, -32.7323) -> (13.6371, -37.4779) centre (21.8863, -42.1897) ccw projected
  line L0 (11.5276, -36.8094) -> (13.6371, -37.4779) projected
  arc A1 (11.5276, -36.8094) -> (10.3193, -40.6226) centre (10.9235, -38.716) ccw projected
  line L1 (12.4289, -41.291) -> (10.3193, -40.6226) projected
  arc A2 (12.4289, -41.291) -> (12.6688, -44.4893) centre (21.8863, -42.1897) ccw projected
  line L2 (11.7586, -44.9612) -> (12.6688, -44.4893) projected
  arc A3 (11.7586, -44.9612) -> (13.7879, -48.8731) centre (21.8863, -42.1897) ccw projected
  line L3 (14.6982, -48.4011) -> (13.7879, -48.8731) projected
  arc A4 (14.6982, -48.4011) -> (17.1744, -50.4389) centre (21.8863, -42.1897) ccw projected
  line L4 (16.506, -52.5484) -> (17.1744, -50.4389) projected
  arc A5 (16.506, -52.5484) -> (20.3191, -53.7567) centre (18.4125, -53.1525) ccw projected
  line L5 (20.9875, -51.6471) -> (20.3191, -53.7567) projected
  arc A6 (20.9875, -51.6471) -> (30.1354, -46.9016) centre (21.8863, -42.1897) ccw projected
  line L6 (32.2449, -47.57) -> (30.1354, -46.9016) projected
  arc A7 (32.2449, -47.57) -> (33.4532, -43.7569) centre (32.8491, -45.6635) ccw projected
  line L7 (31.3437, -43.0884) -> (33.4532, -43.7569) projected
  arc A8 (31.3437, -43.0884) -> (31.1037, -39.8901) centre (21.8863, -42.1897) ccw projected
  line L8 (32.0139, -39.4182) -> (31.1037, -39.8901) projected
  arc A9 (32.0139, -39.4182) -> (29.9846, -35.5064) centre (21.8863, -42.1897) ccw projected
  line L9 (29.0744, -35.9783) -> (29.9846, -35.5064) projected
  arc A10 (29.0744, -35.9783) -> (26.5981, -33.9406) centre (21.8863, -42.1897) ccw projected
  line L10 (27.2666, -31.831) -> (26.5981, -33.9406) projected
  arc A11 (27.2666, -31.831) -> (23.4534, -30.6228) centre (25.36, -31.2269) ccw projected
  line L11 (22.785, -32.7323) -> (23.4534, -30.6228) projected
  line L12 (13.6371, -37.4779) -> (12.4289, -41.291) construction
  line L13 (12.4289, -41.291) -> (8.4128, -40.0184) construction
  line L14 (8.4128, -40.0184) -> (9.621, -36.2053) construction
  line L15 (9.621, -36.2053) -> (13.6371, -37.4779) construction
  line L16 (12.6688, -44.4893) -> (14.6982, -48.4011) construction
  line L17 (14.6982, -48.4011) -> (13.581, -48.9807) construction
  line L18 (13.581, -48.9807) -> (11.5516, -45.0689) construction
  line L19 (11.5516, -45.0689) -> (12.6688, -44.4893) construction
  line L20 (17.1744, -50.4389) -> (20.9875, -51.6471) construction
  line L21 (20.9875, -51.6471) -> (19.715, -55.6632) construction
  line L22 (19.715, -55.6632) -> (15.9018, -54.455) construction
  line L23 (15.9018, -54.455) -> (17.1744, -50.4389) construction
  line L24 (8.1617, -40.1487) -> (12.5591, -41.5421)
  line L25 (12.5591, -41.5421) -> (13.8882, -37.3476)
  line L26 (13.8882, -37.3476) -> (9.4908, -35.9542)
  line L27 (9.4908, -35.9542) -> (8.1617, -40.1487)
  line L28 (11.2146, -44.9621) -> (13.4742, -49.3177)
  line L29 (13.4742, -49.3177) -> (15.0352, -48.5079)
  line L30 (15.0352, -48.5079) -> (12.7756, -44.1523)
  line L31 (12.7756, -44.1523) -> (11.2146, -44.9621)
  line L32 (17.0441, -50.1878) -> (21.2386, -51.5169)
  line L33 (21.2386, -51.5169) -> (19.8452, -55.9143)
  line L34 (19.8452, -55.9143) -> (15.6508, -54.5852)
  line L35 (15.6508, -54.5852) -> (17.0441, -50.1878)
  point P0 (-63.7898, 74.4905)
  dimension "d170" = 0.2
  dimension "d171" = 0.25
  dimension "d172" = 0.2
  constraints: 48 end point, 13 parallel, 6 perpendicular, 9 other
  measures "d170" distance between parallel lines of L13 L24
  measures "d171" distance between parallel lines of L18 L28
  measures "d172" distance between parallel lines of L23 L35
extrude "Extrusion25" cut sketch "Sketch29" against normal up to surface (21.7885 mm away) contours L26 L25 L24 A2 L1 A1 L0 A0 | A0 L0 A1 L1 A2 L24 L27 L26 | L31 L30 L29 A4 L3 A3 L2 A2 | A2 L2 A3 L3 A4 L29 L28 L31 | L35 L32 L33 A6 L5 A5 L4 A4 | A4 L4 A5 L5 A6 L33 L34 L35
fillet "Fillet3" radius 1 4 edges at (-35.4426, -134.894, 11.0794) (-35.4426, -131.7827, 14.1907) (-35.4426, -151.1575, 11.0794) (-35.4426, -154.2687, 14.1907)
move faces "Move1" translate (1.5, 0, 0) faces at (-13.3368, -124.4413, 3.7134)
move faces "Move2" translate (13, 0, 0) faces at (-46.3368, -145.1765, 5.191)
sketch "Sketch30" plane through (0, 0, 2) normal (0, 0, 1) x (1, 0, 0)
  point P0 (0, 0)
sketch "Sketch31" plane through (-93.5594, -157.9139, 2) normal (1, 0, 0) x (0, 0, -1)
  point P0 (2, 157.9139)
sketch "Sketch32" plane through (-93.5594, -157.9139, 2) normal (1, 0, 0) x (0, 0, -1)
  circle A0 centre (-25, 90.627) radius 3.575
  line L0 (-22.6256, 80.627) -> (-15, 88.2526) construction
  line L1 (-15, 93.0014) -> (-22.6256, 100.627) construction
  line L2 (-27.3744, 100.627) -> (-35, 93.0014) construction
  line L3 (-35, 88.2526) -> (-27.3744, 80.627) construction
  line L4 (-30.6938, 76.0415) -> (-21.5025, 99.5863) construction
  line L5 (-19.6712, 80.9474) -> (-24.5756, 89.8562) construction
  line L6 (-30.6938, 76.0415) -> (-2.4168, 76.0415) construction
  line L7 (-35, 88.2526) -> (-35, 93.0014)
  line L8 (-15, 88.2526) -> (-15, 93.0014) construction
  line L9 (-27.3744, 80.627) -> (-22.6256, 80.627) construction
  line L10 (-27.3744, 100.627) -> (-22.6256, 100.627) construction
  circle A1 centre (-25, 90.627) radius 5.2
  line L11 (-35, 0) -> (-35, 155.3673) construction
  line L12 (-35, 90.627) -> (-15, 90.627) construction
  line L13 (-25, 80.627) -> (-25, 100.627) construction
  line L14 (-22.5221, 100.877) -> (-14.75, 93.1049)
  line L15 (-14.75, 93.1049) -> (-14.75, 88.1491)
  line L16 (-14.75, 88.1491) -> (-22.5221, 80.377)
  line L17 (-22.5221, 80.377) -> (-27.4779, 80.377)
  line L18 (-27.4779, 80.377) -> (-35.25, 88.1491)
  line L19 (-35.25, 88.1491) -> (-35.25, 93.1049)
  line L20 (-35.25, 93.1049) -> (-27.4779, 100.877)
  line L21 (-27.4779, 100.877) -> (-22.5221, 100.877)
  line L22 (-28.0992, 78.877) -> (-21.9008, 78.877)
  line L23 (-21.9008, 78.877) -> (-13.25, 87.5278)
  line L24 (-13.25, 87.5278) -> (-13.25, 93.7262)
  line L25 (-13.25, 93.7262) -> (-21.9008, 102.377)
  line L26 (-21.9008, 102.377) -> (-28.0992, 102.377)
  line L27 (-28.0992, 102.377) -> (-36.75, 93.7262)
  line L28 (-36.75, 93.7262) -> (-36.75, 87.5278)
  line L29 (-36.75, 87.5278) -> (-28.0992, 78.877)
  line L30 (-25, 78.877) -> (-25, 85.427)
  line L31 (-25, 95.827) -> (-25, 102.377)
  circle A2 centre (-25, 90.627) radius 5.5
  point P0 (2, 157.9139)
  point P1 (-26.0982, 87.8139)
  point P2 (-22.1234, 85.4018)
  point P3 (-25, 80.377)
  point P4 (-25, 100.877)
  dimension "d182" = 7.15
  dimension "d184" = 45
  dimension "d186" = 17.5
  dimension "d187" = 17.5
  dimension "d188" = 20
  dimension "d189" = 20
  dimension "d190" = 10.4
  dimension "d198" = 0.25
  dimension "d199" = 1.5
  dimension "d204" = 11
  constraints: 62 end point, 11 parallel, 9 midpoint, 5 point on line, 3 centre point, 3 coincident, 3 horizontal, 3 perpendicular, 2 point on circle, 1 vertical, 14 other
  measures "d182" diameter of A0
  measures "d184" angle of L6 L0
  measures "d186" distance between parallel lines of L1 L3
  measures "d187" distance between parallel lines of L0 L2
  measures "d188" distance between parallel lines of L8 L7
  measures "d189" distance between parallel lines of L10 L9
  measures "d190" diameter of A1
  measures "d198" distance between parallel lines of L1 L14
  measures "d199" distance between parallel lines of L17 L22
  measures "d204" diameter of A2
extrude "Extrusion26" cut sketch "Sketch32" against normal through all contours A0
extrude "Extrusion27" add sketch "Sketch32" along normal blind 0.5 contours A1
extrude "Extrusion28" add sketch "Sketch32" along normal blind 3 contours L31 L26 L25 L24 L23 L22 L30 L17 L16 L15 L14 L21
extrude "Extrusion29" add sketch "Sketch32" along normal blind 1.5 from surface at 3 contours A1 L31 A2 L30 | L31 L21 L14 L15 L16 L17 L30 A2 | L31 L26 L25 L24 L23 L22 L30 L17 L16 L15 L14 L21 picked at (-23.4109, 85.498)
sketch "Sketch33" plane through (-76.3368, -95.497, 22.3224) normal (-1, 0, 0) x (0, -0.4604848, 0.8876676)
  line L0 (2.9103, -4.1418) -> (1.5185, -1.4556)
  circle A0 centre (2.9103, -4.1418) radius 1
  circle A1 centre (16.2343, -29.865) radius 1
  line L1 (3.1465, -4.5939) -> (1.5185, -1.4556) projected
  arc A2 (3.1465, -4.5939) -> (16.0254, -29.4204) centre (8.9946, -17.3139) ccw projected
  line L2 (3.7982, -3.6818) -> (2.0318, -4.6195) construction
  line L3 (17.1219, -29.4044) -> (15.3554, -30.3421) construction
  point P0 (-63.7898, 74.4905)
  dimension "d205" = 2
  dimension "d206" = 2
  dimension "d209" = 0.5
  dimension "d210" = 0.5
  constraints: 6 end point, 4 point on circle, 2 centre point, 1 parallel
  measures "d205" diameter of A0
  measures "d206" diameter of A1
  measures "d209" distance from line of A2.end L3
  measures "d210" distance from line of L1.start L2
extrude "Extrusion30" add sketch "Sketch33" against normal up to surface (30 mm away)